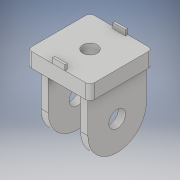
# Autodesk Inventor part: item_gelenk_teil_laengs
Saved by Autodesk Inventor 2018 (Build 220112000, 112)
## iProperties
Created: 2020-04-19
Part Number: item_gelenk_teil_laengs
Material: Generisch
Document SubType Name: Modeling
Designer: wepet
Density: 1 g/cm^3
Appearance: Vorgabe
Author: wepet
Autodesk Inventor part; units mm, degrees
ref_plane "YZ Plane" through (0, 0, 0) normal (1, 0, 0) x (0, 1, 0)
ref_plane "XZ Plane" through (0, 0, 0) normal (0, 1, 0) x (-1, 0, 0)
ref_plane "XY Plane" through (0, 0, 0) normal (0, 0, 1) x (1, 0, 0)
sketch "Skizze1" plane through (0, 0, 0) normal (0, 0, 1) x (1, 0, 0)
  line L0 (0.2, 0) -> (2.8, 0)
  line L1 (3, 0.2) -> (3, 2.8)
  line L2 (2.8, 3) -> (0.2, 3)
  line L3 (0, 2.8) -> (0, 0.2)
  arc A0 (0.2, 3) -> (0, 2.8) centre (0.2, 2.8) ccw
  arc A1 (3, 2.8) -> (2.8, 3) centre (2.8, 2.8) ccw
  arc A2 (2.8, 0) -> (3, 0.2) centre (2.8, 0.2) ccw
  arc A3 (0, 0.2) -> (0.2, 0) centre (0.2, 0.2) ccw
  line L4 (0, 1.5) -> (3, 1.5) construction
  line L5 (1.5, 3) -> (1.5, 0) construction
  circle A4 centre (1.5, 1.5) radius 0.35
  point P0 (0, 0)
  point P1 (3, 3)
  point P2 (3, 0)
  point P3 (0, 3)
  dimension "d0" = 3
  dimension "d1" = 3
  dimension "d2" = 0.2
  dimension "d3" = 0.7
  constraints: 12 end point, 8 point on circle, 8 point on line, 8 tangent, 5 centre point, 5 midpoint, 3 equal radius, 2 parallel, 1 horizontal, 1 perpendicular
  measures "d0" distance of point (0, 3) point (3, 3)
  measures "d1" distance of point (3, 3) point (3, 0)
  measures "d2" radius of A0
  measures "d3" diameter of A4
extrude "Extrusion1" add sketch "Skizze1" along normal blind 0.7
sketch "Skizze2" plane through (0, 0, 0.7) normal (0, 0, 1) x (1, 0, 0)
  circle A0 centre (1.5, 1.5) radius 0.35 construction
  line L0 (2.8, 3) -> (0.2, 3) construction
  arc A1 (0.2, 3) -> (0, 2.8) centre (0.2, 2.8) ccw construction
  line L1 (0, 2.8) -> (0, 0.2) construction
  arc A2 (0, 0.2) -> (0.2, 0) centre (0.2, 0.2) ccw construction
  line L2 (0.2, 0) -> (2.8, 0) construction
  arc A3 (2.8, 0) -> (3, 0.2) centre (2.8, 0.2) ccw construction
  line L3 (3, 0.2) -> (3, 2.8) construction
  arc A4 (3, 2.8) -> (2.8, 3) centre (2.8, 2.8) ccw construction
  line L4 (0, 2.8) -> (0, 0.2) projected
  line L5 (0, 1.8) -> (0.1, 1.8)
  line L6 (0.1, 1.8) -> (0.1, 1.2)
  line L7 (0.1, 1.2) -> (0, 1.2)
  line L8 (0, 1.2) -> (0, 1.8)
  line L9 (0.2, 0) -> (2.8, 0) projected
  line L10 (1.2, 0) -> (1.8, 0)
  line L11 (1.8, 0) -> (1.8, 0.1)
  line L12 (1.8, 0.1) -> (1.2, 0.1)
  line L13 (1.2, 0.1) -> (1.2, 0)
  line L14 (3, 0.2) -> (3, 2.8) projected
  line L15 (3, 1.2) -> (2.9, 1.2)
  line L16 (2.9, 1.2) -> (2.9, 1.8)
  line L17 (2.9, 1.8) -> (3, 1.8)
  line L18 (3, 1.8) -> (3, 1.2)
  line L19 (0.2, 3) -> (2.8, 3) projected
  line L20 (1.8, 3) -> (1.2, 3)
  line L21 (1.2, 3) -> (1.2, 2.9)
  line L22 (1.2, 2.9) -> (1.8, 2.9)
  line L23 (1.8, 2.9) -> (1.8, 3)
  point P0 (0, 0)
  point P1 (0, 1.5)
  point P2 (1.5, 3)
  point P3 (1.5, 0)
  dimension "d6" = 0.6
  dimension "d7" = 0.1
  dimension "d8" = 0.6
  dimension "d9" = 0.6
  dimension "d10" = 0.6
  dimension "d11" = 0.1
  dimension "d12" = 0.1
  dimension "d13" = 0.1
  constraints: 32 end point, 8 parallel, 6 midpoint, 4 horizontal, 4 perpendicular, 4 point on line
  measures "d6" distance of L5.end L6.end
  measures "d7" distance of L5.start L5.end
  measures "d8" distance of L21.end L22.end
  measures "d9" distance of L15.end L16.end
  measures "d10" distance of L11.end L12.end
  measures "d11" distance of L22.end L20.start
  measures "d12" distance of L16.end L17.end
  measures "d13" distance of L10.end L11.end
extrude "Extrusion2" add sketch "Skizze2" along normal blind 0.25 separate body contours L13 L12 L11 L9 | L19 L23 L22 L21
sketch "Skizze3" plane through (0, 0, 0) normal (0, 0, -1) x (-1, 0, 0)
  circle A0 centre (-1.5, 1.5) radius 0.35 construction
  line L0 (-0.2, 3) -> (-2.8, 3) construction
  arc A1 (-2.8, 3) -> (-3, 2.8) centre (-2.8, 2.8) ccw construction
  line L1 (-3, 2.8) -> (-3, 0.2) construction
  arc A2 (-3, 0.2) -> (-2.8, 0) centre (-2.8, 0.2) ccw construction
  line L2 (-2.8, 0) -> (-0.2, 0) construction
  arc A3 (-0.2, 0) -> (0, 0.2) centre (-0.2, 0.2) ccw construction
  line L3 (0, 0.2) -> (0, 2.8) construction
  arc A4 (0, 2.8) -> (-0.2, 3) centre (-0.2, 2.8) ccw construction
  line L4 (-2.8, 2.9) -> (-2.45, 2.9)
  line L5 (-2.45, 2.9) -> (-2.45, 0.1)
  line L6 (-2.45, 0.1) -> (-2.8, 0.1)
  line L7 (-2.8, 0.1) -> (-2.8, 2.9)
  line L8 (-0.9, 2.9) -> (-0.55, 2.9)
  line L9 (-0.55, 2.9) -> (-0.55, 0.1)
  line L10 (-0.55, 0.1) -> (-0.9, 0.1)
  line L11 (-0.9, 0.1) -> (-0.9, 2.9)
  line L12 (-3, 1.5) -> (0, 1.5) construction
  point P0 (0, 0)
  point P1 (-2.8, 1.5)
  dimension "d16" = 0.35
  dimension "d17" = 0.35
  dimension "d18" = 2.8
  dimension "d19" = 0.2
  dimension "d20" = 0.55
  constraints: 18 end point, 4 parallel, 3 midpoint, 3 point on line, 2 horizontal, 2 perpendicular
  measures "d16" distance of L4.start L4.end
  measures "d17" distance of L8.start L8.end
  measures "d18" distance of L6.end L4.start
  measures "d19" distance between parallel lines of L7 L1
  measures "d20" distance between parallel lines of L3 L9
extrude "Extrusion3" add sketch "Skizze3" along normal blind 1.55 bodies 1
sketch "Skizze4" plane through (2.8, 0.1, 0) normal (1, 0, 0) x (0, 0, -1)
  line L0 (1.55, 2.8) -> (1.55, 0) projected
  line L1 (1.55, 2.8) -> (1.55, 0) construction
  arc A0 (1.55, 0) -> (1.55, 2.8) centre (1.55, 1.4) ccw
  point P0 (0, -0.1)
  constraints: 2 end point, 2 point on circle, 1 centre point, 1 midpoint
extrude "Extrusion4" add sketch "Skizze4" against normal blind 0.35 bodies 1
sketch "Skizze5" plane through (0.55, 0.1, 0) normal (-1, 0, 0) x (0, 0, 1)
  line L0 (-1.55, 0) -> (-1.55, 2.8) projected
  arc A0 (-1.55, 2.8) -> (-1.55, 0) centre (-1.55, 1.4) ccw projected
  point P0 (0, -0.1)
extrude "Extrusion5" add sketch "Skizze5" against normal blind 0.35 bodies 1
sketch "Skizze6" plane through (0.55, 0.1, 0) normal (-1, 0, 0) x (0, 0, 1)
  arc A0 (-1.55, 2.8) -> (-1.55, 0) centre (-1.55, 1.4) ccw construction
  point P0 (0, -0.1)
  dimension "d6" = 0.6
  dimension "d7" = 0.1
  constraints: 1 coincident
hole "Bohrung1" at (0.55, 1.5, -1.55) direction (1, 0, 0) diameter 0.8 end through all bodies 1
